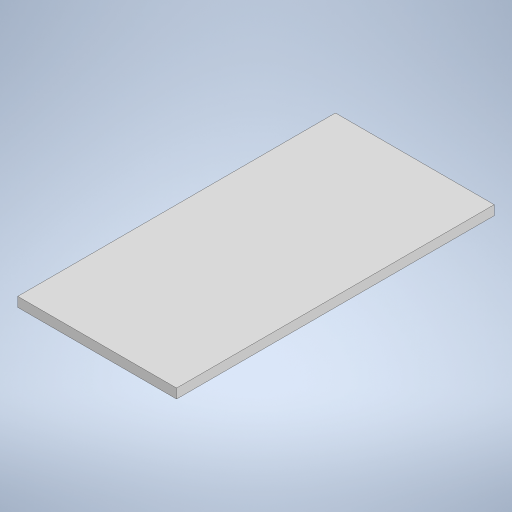
# Autodesk Inventor part: Basis of the robot
Saved by Autodesk Inventor 2023 (Build 270158000, 158)
## iProperties
Created: 2023-05-15
Part Number: Basis of the robot
Material: Типовые
Document SubType Name: Modeling
Designer: ivanc
Density: 1 g/cm^3
Appearance: По умолчанию
Author: ivanc
Autodesk Inventor part; units mm, degrees
ref_plane "YZ Plane" through (0, 0, 0) normal (1, 0, 0) x (0, 1, 0)
ref_plane "XZ Plane" through (0, 0, 0) normal (0, 1, 0) x (-1, 0, 0)
ref_plane "XY Plane" through (0, 0, 0) normal (0, 0, 1) x (1, 0, 0)
sketch "Эскиз1" plane through (0, 0, 0) normal (0, 1, 0) x (-1, 0, 0)
  line L0 (-25, 50) -> (25, 50)
  line L1 (25, 50) -> (25, -50)
  line L2 (25, -50) -> (-25, -50)
  line L3 (-25, -50) -> (-25, 50)
  line L4 (-25, 50) -> (25, -50) construction
  line L5 (25, 50) -> (-25, -50) construction
  point P0 (0, 0)
  dimension "d0" = 50
  dimension "d1" = 100
  constraints: 12 end point, 2 midpoint, 2 parallel, 1 horizontal, 1 perpendicular
  measures "d0" distance of L1.end L2.end
  measures "d1" distance of L0.end L1.end
extrude "Выдавливание1" add sketch "Эскиз1" along normal blind 3
